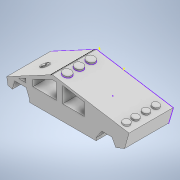
# Autodesk Inventor part: truck body
Saved by Autodesk Inventor 2021 (Build 250183000, 183)
## iProperties
Created: 2021-07-03
Part Number: truck body
Material: Generic
Document SubType Name: Modeling
Designer: USER
Density: 1 g/cm^3
Appearance: Default
Author: USER
Autodesk Inventor part; units mm, degrees
ref_plane "YZ Plane" through (0, 0, 0) normal (1, 0, 0) x (0, 1, 0)
ref_plane "XZ Plane" through (0, 0, 0) normal (0, 1, 0) x (-1, 0, 0)
ref_plane "XY Plane" through (0, 0, 0) normal (0, 0, 1) x (1, 0, 0)
sketch "Sketch1" plane through (0, 0, 0) normal (0, 0, 1) x (1, 0, 0)
  line L0 (-21.2308, 0.5024) -> (-22.7161, 0.9392)
  line L1 (-22.7161, 0.9392) -> (-23.1093, 3.2982)
  line L2 (-23.1093, 3.2982) -> (-7.6012, 11.5983)
  line L3 (-7.6012, 11.5983) -> (18.4787, 7.4483)
  line L4 (18.4787, 7.4483) -> (16.9112, 2.1187)
  line L5 (16.9112, 2.1187) -> (13.9355, 0.9392)
  line L6 (13.9355, 0.9392) -> (12.6303, 3.3778)
  line L7 (12.6303, 3.3778) -> (9.1738, 3.3778)
  line L8 (9.1738, 3.3778) -> (7.2578, 0.5024)
  line L9 (7.2578, 0.5024) -> (7.2578, -0.415)
  line L10 (7.2578, -0.415) -> (-15.3552, -0.415)
  line L11 (-15.3552, -0.415) -> (-15.3552, 0.5024)
  line L12 (-15.3552, 0.5024) -> (-16.4949, 3.3778)
  line L13 (-16.4949, 3.3778) -> (-20.3851, 3.3778)
  line L14 (-20.3851, 3.3778) -> (-21.2308, 0.5024)
  line L15 (-19.3524, 4.7835) -> (-7.6012, 11.0729)
  line L16 (-7.6012, 11.0729) -> (4.0011, 9.2266)
  line L17 (4.0011, 9.2266) -> (3.8573, -0.415)
  line L18 (-19.3524, 4.7835) -> (-14.1976, 4.7835)
  line L19 (-14.1976, 4.7835) -> (-14.1976, -0.415)
  line L20 (-5.6947, 10.7695) -> (-5.6947, -0.415)
  line L21 (-4.8279, 10.6316) -> (-4.8279, -0.415)
  line L22 (-14.1976, 6.9677) -> (-7.7481, 10.1497)
  line L23 (-7.7481, 10.1497) -> (-6.1966, 10.1497)
  line L24 (-6.1966, 10.1497) -> (-6.1966, 4.7835)
  line L25 (-6.1966, 4.7835) -> (-14.1976, 4.7835)
  line L26 (-14.1976, 6.9677) -> (-14.1976, 4.7835)
  line L27 (-4.1011, 10.1737) -> (3.2727, 9.0003)
  line L28 (3.2727, 9.0003) -> (3.2727, 4.7835)
  line L29 (3.2727, 4.7835) -> (-4.1011, 4.7835)
  line L30 (-4.1011, 4.7835) -> (-4.1011, 10.1737)
  point P0 (0, 0)
  constraints: 62 end point, 14 perpendicular, 9 point on line, 4 parallel, 2 horizontal, 1 vertical
extrude "Extrusion1" add sketch "Sketch1" along normal blind 15 contours L0 L1 L2 L3 L4 L5 L6 L7 L8 L9 L10 L17 L16 L15 L18 L19 L11 L12 L13 L14 | L26 L22 L23 L24 L25 | L19 L18 L15 L16 L20 L10 | L20 L16 L21 L10 | L21 L16 L17 L10 | L27 L28 L29 L30
sketch "Sketch2" plane through (0, 0, 15) normal (0, 0, 1) x (1, 0, 0)
  line L0 (-19.0429, 4.7716) -> (-16.5922, 6.0833)
  line L1 (-7.6012, 11.5983) -> (-23.1093, 3.2982) projected
  line L2 (-16.5922, 6.0833) -> (-16.5922, 4.7716)
  line L3 (-16.5922, 4.7716) -> (-19.0429, 4.7716)
  point P0 (0, 0)
  constraints: 6 end point, 1 parallel, 1 perpendicular, 1 point on line, 1 vertical
extrude "Extrusion2" cut sketch "Sketch2" against normal through all both and the other way through all
extrude "Extrusion3" cut sketch "Sketch1" along normal through all contours L26 L22 L23 L24 L25
extrude "Extrusion4" cut sketch "Sketch1" along normal through all contours L27 L28 L29 L30
sketch "Sketch3" plane through (-7.6012, 11.5983, 15) normal (0.1571517, 0.9875745, 0) x (0.9875745, -0.1571517, 0)
  point P0 (9.3294, 15)
sketch "Sketch4" plane through (-7.6012, 11.5983, 15) normal (0.1571517, 0.9875745, 0) x (0.9875745, -0.1571517, 0)
  point P0 (9.3294, 15)
  point P1 (14.4418, 6.2264)
sketch "Sketch5" plane through (-23.1093, 3.2982, 15) normal (-0.4718768, 0.8816645, 0) x (0.8816645, 0.4718768, 0)
  line L0 (16.7765, 15) -> (16.7765, 0) projected
  line L1 (16.7765, 15) -> (16.7765, 0)
  point P0 (18.8183, 15)
  constraints: 2 end point, 1 collinear
sketch "Sketch12" plane through (-7.6012, 11.5983, 15) normal (0.1571517, 0.9875745, 0) x (0.9875745, -0.1571517, 0)
  circle A0 centre (23.4582, 1.9446) radius 1.1665
  circle A1 centre (23.4582, 5.0462) radius 1.1665
  circle A2 centre (23.4582, 8.5859) radius 1.1665
  circle A3 centre (23.4582, 11.9232) radius 1.1665
  line L0 (22.1103, 0.3163) -> (24.9814, 0.3163)
  line L1 (24.9814, 0.3163) -> (24.9814, 13.9844)
  line L2 (24.9814, 13.9844) -> (22.1103, 13.9844)
  line L3 (22.1103, 13.9844) -> (22.1103, 0.3163)
  point P0 (9.3294, 15)
  constraints: 8 end point, 4 centre point, 2 parallel, 1 horizontal, 1 perpendicular
sketch "Sketch13" plane through (-7.6012, 11.5983, 15) normal (0.1571517, 0.9875745, 0) x (0.9875745, -0.1571517, 0)
  point P0 (9.3294, 15)
extrude "Extrusion11" add sketch "Sketch12" along normal blind 0.5 contours A0 | A1 | A2 | A3
sketch "Sketch14" plane through (-7.6012, 11.5983, 15) normal (0.1571517, 0.9875745, 0) x (0.9875745, -0.1571517, 0)
  line L0 (23.5, 2.1302) -> (23.5, 2.0843)
  line L1 (23.5, 2.0843) -> (23.5, 1.9717)
  point P0 (9.3294, 15)
  constraints: 4 end point, 1 vertical
sketch "Sketch15" plane through (-7.6012, 11.5983, 15) normal (0.1571517, 0.9875745, 0) x (0.9875745, -0.1571517, 0)
  circle A0 centre (2, 3) radius 1.4142
  circle A1 centre (2, 11) radius 1.414
  circle A2 centre (2, 7) radius 1.414
  point P0 (9.3294, 15)
  constraints: 3 centre point
extrude "Extrusion12" add sketch "Sketch15" along normal blind 0.5
sketch "Sketch16" plane through (-23.1093, 3.2982, 15) normal (-0.4718768, 0.8816645, 0) x (0.8816645, 0.4718768, 0)
  circle A0 centre (8, 6) radius 1.4142
  point P0 (18.8183, 15)
  constraints: 1 centre point
sketch "Sketch17" plane through (-23.1093, 3.2982, 15) normal (-0.4718768, 0.8816645, 0) x (0.8816645, 0.4718768, 0)
  point P0 (18.8183, 15)
extrude "Extrusion13" add sketch "Sketch16" along normal blind 0.25
sketch "Sketch18" plane through (-16.1739, 7.2936, 9) normal (-0.4718768, 0.8816645, 0) x (0.8816645, 0.4718768, 0)
  point P0 (10.8183, 9)
sketch "Sketch19" plane through (-16.1739, 7.2936, 9) normal (-0.4718768, 0.8816645, 0) x (0.8816645, 0.4718768, 0)
  point P0 (10.8183, 9)
sketch "Sketch20" plane through (-16.1739, 7.2936, 9) normal (-0.4718768, 0.8816645, 0) x (0.8816645, 0.4718768, 0)
  line L0 (0.1686, 1.1782) -> (-0.9399, 0.7449) construction
  line L1 (-0.9399, 0.7449) -> (0, 0) construction
  line L2 (0, 0) -> (1, 0) construction
  line L3 (1, 0) -> (0, -1) construction
  line L4 (0, -1) -> (-0.5704, -0.7197) construction
  spline S0 degree 4 poles (0.1686, 1.1782) (-0.9399, 0.7449) (0, 0) (1, 0) (0, -1) (-0.5704, -0.7197) knots 1 1 1 1 1 2 3 3 3 3 3
  line L5 (0.1686, 1.1782) -> (-0.2137, 0.6958) construction
  line L6 (-0.2137, 0.6958) -> (1, 0) construction
  line L7 (1, 0) -> (0.737, -0.263) construction
  line L8 (0.737, -0.263) -> (0.3757, -0.9696) construction
  line L9 (0.3757, -0.9696) -> (-0.1384, -1.1517) construction
  line L10 (-0.1384, -1.1517) -> (-0.5704, -0.7197) construction
  spline S1 degree 4 poles (0.1686, 1.1782) (-0.2137, 0.6958) (1, 0) (0.737, -0.263) (0.3757, -0.9696) (-0.1384, -1.1517) (-0.5704, -0.7197) knots 1 1 1 1 1 2 3 4 4 4 4 4
  point P0 (10.8183, 9)
  constraints: 1 coincident, 1 perpendicular, 1 point on line, 6 other
extrude "Extrusion14" cut sketch "Sketch20" against normal blind 0.25
sketch "Sketch21" plane through (15.6442, 8.4056, 13.0554) normal (0.1571517, 0.9875745, 0) x (0.9875745, -0.1571517, 0)
  point P0 (-14.1288, 13.0554)
sketch "Sketch22" plane through (-5.5474, 11.7778, 12) normal (0.1571517, 0.9875745, 0) x (0.9875745, -0.1571517, 0)
  point P0 (7.3294, 12)
body "Solid1"
